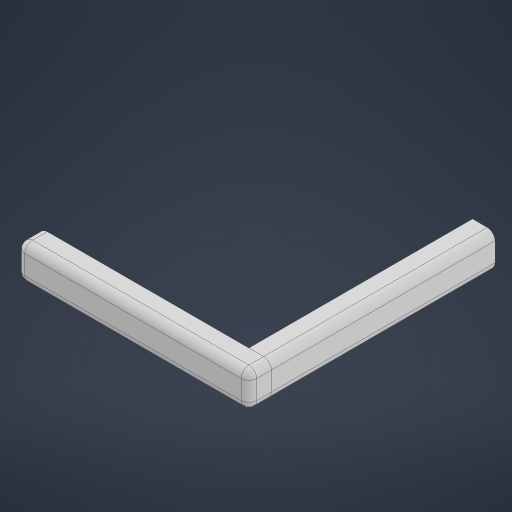
# Autodesk Inventor part: Bumper
Saved by Autodesk Inventor 2023 (Build 270158000, 158)
## iProperties
Created: 2023-01-12
Part Number: Bumper
Material: Generic
Document SubType Name: Modeling
Designer: Blank Slate
Density: 1 g/cm^3
Appearance: Default
Author: Blank Slate
Autodesk Inventor part; units mm, degrees
ref_plane "YZ Plane" through (0, 0, 0) normal (1, 0, 0) x (0, 1, 0)
ref_plane "XZ Plane" through (0, 0, 0) normal (0, 1, 0) x (-1, 0, 0)
ref_plane "XY Plane" through (0, 0, 0) normal (0, 0, 1) x (1, 0, 0)
sketch "Sketch1" plane through (0, 0, 0) normal (1, 0, 0) x (0, 1, 0)
  line L0 (0, 0) -> (127, 0)
  line L1 (127, 0) -> (127, 82.55)
  line L2 (127, 82.55) -> (0, 82.55)
  line L3 (0, 82.55) -> (0, 0)
  dimension "d0" = 127
  dimension "d1" = 82.55
  constraints: 8 end point, 2 parallel, 1 horizontal, 1 perpendicular
  measures "d0" distance of L2.end L1.end
  measures "d1" distance of L1.end L0.end
extrude "Extrusion1" add sketch "Sketch1" along normal blind 850.9
sketch "Sketch2" plane through (0, 0, 0) normal (0, 0, -1) x (-1, 0, 0)
  line L0 (-850.9, 127) -> (-768.35, 127)
  line L1 (-768.35, 127) -> (-768.35, 0)
  line L2 (-768.35, 0) -> (-850.9, 0)
  line L3 (-850.9, 0) -> (-850.9, 127)
  point P0 (0, 0)
  dimension "d8" = 82.55
  dimension "d9" = 127
  constraints: 8 end point, 2 parallel, 1 horizontal, 1 perpendicular
  measures "d8" distance of L1.end L2.end
  measures "d9" distance of L0.end L1.end
extrude "Extrusion2" add sketch "Sketch2" along normal blind 820.674 separate body
fillet "Fillet1" radius 28.575 10 edges at (425.45, 127, 82.55) (425.45, 0, 82.55) (850.9, 127, 41.275) (850.9, 0, 41.275) (850.9, 63.5, 82.55) (0, 63.5, 82.55) (0, 127, 41.275) (0, 0, 41.275) (850.9, 127, -410.337) (850.9, 0, -410.337)
body "Solid1"
body "Solid2"
